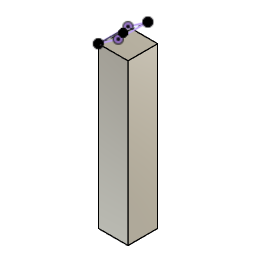
Finger Sim MASTER F3Z (Autodesk Fusion 360 archive; units mm, degrees)
design "Rod"
Autodesk Fusion 360 part; units mm, degrees
sketch "Sketch1" plane through (0, 0, 0) normal (0, 0, 1) x (1, 0, 0)
  line L0 (3.175, 3.175) -> (-3.175, 3.175)
  line L1 (-3.175, 3.175) -> (-3.175, -3.175)
  line L2 (-3.175, -3.175) -> (3.175, -3.175)
  line L3 (3.175, -3.175) -> (3.175, 3.175)
  line L4 (3.175, 3.175) -> (-3.175, -3.175) construction
  line L5 (-3.175, 3.175) -> (3.175, -3.175) construction
  dimension "d1" = 6.35
  dimension "d2" = 6.35
  constraint horizontal L0
  constraint perpendicular L0 L1
  constraint parallel L0 L2
  constraint parallel L1 L3
  constraint coincident L4 origin
  constraint coincident L5 origin
  measures "d1" distance of L1.end L2.end
  measures "d2" distance of L0.end L1.end
extrude "Extrude1" add sketch "Sketch1" along normal blind 45.72
ref_plane "WorkPlane1" through (-3.175, 0, 45.72) normal (-0.573576, 0, 0.819152) x (0, -1, 0)
sketch "Sketch2" plane through (-22.5259, 0, 32.1703) normal (-0.573576, 0, 0.819152) x (0, -1, 0)
  line L0 (3.175, 28.8247) -> (-3.175, 28.8247)
  line L1 (-3.175, 28.8247) -> (-3.175, 23.6231)
  line L2 (-3.175, 23.6231) -> (3.175, 23.6231)
  line L3 (3.175, 23.6231) -> (3.175, 28.8247)
  line L4 (-3.175, 28.8247) -> (3.175, 23.6231) construction
  point P0 (0, 26.2239)
  constraint coincident L0.end L1.start
  constraint coincident L2.end L3.start
  constraint midpoint L4 P0
extrude "Extrude2" cut 1 faces at (-1.0583, -1.0583, 0) along direction (0, 0, 1) blind 11.43
